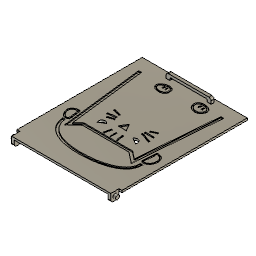
盖子 (Autodesk Fusion 360 design; units mm, degrees)
part number: 2025-10-22-10-29-16-926
Autodesk Fusion 360 part; units mm, degrees
sketch "Sketch1" plane through (0, 0, 0) normal (0, 0, 1) x (1, 0, 0)
  line L0 (50.828, 64.624) -> (-50.828, 64.624)
  line L1 (-50.828, 64.624) -> (-50.828, -64.624)
  line L2 (-50.828, -64.624) -> (50.828, -64.624)
  line L3 (50.828, -64.624) -> (50.828, 64.624)
  line L4 (50.828, 64.624) -> (-50.828, -64.624) construction
  line L5 (-50.828, 64.624) -> (50.828, -64.624) construction
  dimension "d1" = 101.656
  dimension "d2" = 129.248
  constraint horizontal L0
  constraint perpendicular L0 L1
  constraint parallel L0 L2
  constraint parallel L1 L3
  constraint coincident L4 origin
  constraint coincident L5 origin
  measures "d1" distance of L1.end L2.end
  measures "d2" distance of L0.end L1.end
extrude "Extrude1" add sketch "Sketch1" along normal blind 2
sketch "Sketch2" plane through (0, 0, 2) normal (0, 0, 1) x (-1, 0, 0)
  line L0 (-50.828, 64.624) -> (-50.828, -64.624)
  line L1 (-50.828, -64.624) -> (50.828, -64.624)
  line L2 (50.828, -64.624) -> (50.828, 64.624)
  line L3 (50.828, 64.624) -> (-50.828, 64.624)
  line L4 (0, 64.624) -> (0, -64.624) construction
  line L5 (-50.828, 64.624) -> (-48, 64.624) construction
  line L6 (-48, 64.624) -> (-48, 56.624)
  line L7 (-48, 56.624) -> (-50.828, 56.624)
  line L8 (-50.828, 56.624) -> (-50.828, 64.624) construction
  dimension "d5" = 2.828
  dimension "d6" = 8
  constraint midpoint L3 L4.start
  constraint midpoint L1 L4.end
  constraint horizontal L5
  constraint vertical L6
  constraint horizontal L7
  constraint vertical L8
  constraint coincident L0.start L3.end
  measures "d5" distance of L0.start L5.end
  measures "d6" distance of L0.start L7.end
extrude "Extrude2" cut sketch "Sketch2" against normal blind 2 contours L0 L3 L6 L7
mirror "Mirror1" about plane through (0, 0, 0) normal (1, 0, 0) of "Extrude2"
sketch "Sketch3" plane through (0, 0, 0) normal (0, 0, -1) x (1, 0, 0)
  line L0 (-48, 64.624) -> (-48, 56.624)
  line L1 (-48, 56.624) -> (-50.828, 56.624)
  line L2 (-50.828, 56.624) -> (-50.828, -64.624)
  line L3 (-50.828, -64.624) -> (50.828, -64.624)
  line L4 (50.828, -64.624) -> (50.828, 56.624)
  line L5 (50.828, 56.624) -> (48, 56.624)
  line L6 (48, 56.624) -> (48, 64.624)
  line L7 (48, 64.624) -> (-48, 64.624)
  line L8 (48, 56.624) -> (-48, 56.624)
  line L9 (-48, 56.624) -> (-48, 64.624)
  line L10 (-48, 64.624) -> (48, 64.624)
  line L11 (48, 64.624) -> (48, 56.624)
  constraint horizontal L8
  constraint vertical L9
  constraint horizontal L10
  constraint vertical L11
  constraint coincident L0.start L7.end
  constraint coincident L5.end L6.start
extrude "Extrude3" add sketch "Sketch3" along normal blind 6 contours L0 L6 L7 L8 L9 L10 L11
fillet "Fillet1" radius 2 2 edges at (0, -64.624, -6) (0, -56.624, -6)
sketch "Sketch4" plane through (48, 0, 0) normal (1, 0, 0) x (0, 1, 0)
  line L0 (-56.624, 2) -> (-64.624, 2)
  line L1 (-64.624, 2) -> (-64.624, -4)
  line L2 (-62.624, -6) -> (-58.624, -6)
  line L3 (-56.624, -4) -> (-56.624, 0)
  line L4 (-56.624, 0) -> (-56.624, 2)
  circle A0 centre (-60.624, -2) radius 1.995
  arc A1 (-58.624, -6) -> (-56.624, -4) centre (-58.624, -4) ccw
  arc A2 (-64.624, -4) -> (-62.624, -6) centre (-62.624, -4) ccw
  dimension "d13" = 3.99
  measures "d13" diameter of A0
extrude "Extrude4" add sketch "Sketch4" along normal blind 2.5 contours A0
sketch "Sketch5" plane through (0, 0, -6) normal (0, 0, -1) x (1, 0, 0)
  line L0 (-48, 62.624) -> (-48, 58.624)
  line L1 (48, 58.624) -> (48, 62.624)
  line L2 (45.3194, 56.624) -> (-45.3194, 56.624)
  line L3 (-45.3194, 56.624) -> (-45.3194, 65.376)
  line L4 (-45.3194, 65.376) -> (45.3194, 65.376)
  line L5 (45.3194, 65.376) -> (45.3194, 56.624)
  line L6 (45.3194, 56.624) -> (-45.3194, 65.376) construction
  line L7 (-45.3194, 56.624) -> (45.3194, 65.376) construction
  line L8 (-48, 58.624) -> (48, 58.624)
  line L9 (48, 62.624) -> (-48, 62.624)
  point P0 (0, 61)
  constraint horizontal L2
  constraint perpendicular L2 L3
  constraint parallel L2 L4
  constraint parallel L3 L5
  constraint coincident L6 P0
  constraint coincident L7 P0
extrude "Extrude5" cut sketch "Sketch5" against normal blind 6 contours L2 L3 L5 L8
mirror "Mirror2" about plane through (0, 0, 0) normal (1, 0, 0) of "Extrude4"
sketch "Sketch6" plane through (0, 0, -6) normal (0, 0, -1) x (1, 0, 0)
  line L0 (45.3194, 58.624) -> (48, 58.624)
  line L1 (48, 58.624) -> (48, 62.624)
  line L2 (48, 62.624) -> (-48, 62.624)
  line L3 (-48, 62.624) -> (-48, 58.624)
  line L4 (-48, 58.624) -> (-45.3194, 58.624)
  line L5 (-45.3194, 58.624) -> (45.3194, 58.624)
  line L6 (45.3194, 58.624) -> (-45.3194, 58.624)
  line L7 (-45.3194, 58.624) -> (-45.3194, 66.624)
  line L8 (-45.3194, 66.624) -> (45.3194, 66.624)
  line L9 (45.3194, 66.624) -> (45.3194, 58.624)
  line L10 (45.3194, 58.624) -> (-45.3194, 66.624) construction
  line L11 (-45.3194, 58.624) -> (45.3194, 66.624) construction
  point P0 (0, 62.624)
  constraint horizontal L6
  constraint perpendicular L6 L7
  constraint parallel L6 L8
  constraint parallel L7 L9
  constraint coincident L10 P0
  constraint coincident L11 P0
  constraint coincident L0.start L5.end
  constraint midpoint L2 P0
extrude "Extrude6" cut sketch "Sketch6" against normal blind 6 contours L2 L5 L6 L7 L9 | L2 L7 L8 L9
sketch "Sketch7" plane through (0, 0, 2) normal (0, 0, 1) x (-1, 0, 0)
  line L0 (48, 56.624) -> (48, 64.624)
  line L1 (48, 64.624) -> (-48, 64.624)
  line L2 (-48, 64.624) -> (-48, 56.624)
  line L3 (-48, 56.624) -> (-50.828, 56.624)
  line L4 (-50.828, 56.624) -> (-50.828, -64.624)
  line L5 (-50.828, -64.624) -> (50.828, -64.624)
  line L6 (50.828, -64.624) -> (50.828, 56.624)
  line L7 (50.828, 56.624) -> (48, 56.624)
  line L8 (-39.5943, -52.7414) -> (-32.6577, 29.4135)
  line L9 (-32.6577, 29.4135) -> (-22.0361, 21.1764)
  line L10 (-22.0361, 21.1764) -> (23.0515, 21.1764)
  line L11 (23.0515, 21.1764) -> (31.7222, 29.4135)
  line L12 (31.7222, 29.4135) -> (41.26, -51.4408)
  line L13 (-36.9696, -52.963) -> (-30.4409, 24.361)
  line L14 (-30.4409, 24.361) -> (-22.9378, 18.5423)
  line L15 (-22.9378, 18.5423) -> (24.1033, 18.5423)
  line L16 (24.1033, 18.5423) -> (29.7226, 23.8806)
  line L17 (29.7226, 23.8806) -> (38.6441, -51.7494)
  line L18 (-39.5943, -52.7414) -> (-36.9696, -52.963)
  line L19 (38.6441, -51.7494) -> (41.26, -51.4408)
  line L20 (-2.9359, 4.5075) -> (5, 4.5075)
  line L21 (5, 4.5075) -> (1.0321, -2.1031)
  line L22 (1.0321, -2.1031) -> (-2.9359, 4.5075)
  line L23 (-18.3094, 10.9644) -> (-12.3137, 7.7359)
  line L24 (12.7451, 8.0434) -> (18.2795, 11.4256)
  arc A0 (-18.3094, 10.9644) -> (-12.3137, 7.7359) centre (-15.3116, 9.3501) ccw
  arc A1 (12.7451, 8.0434) -> (18.2795, 11.4256) centre (15.5123, 9.7345) ccw
  line L25 (-22.8155, 3.2022) -> (-12.8166, -0.1308)
  line L26 (-21.9822, -3.4637) -> (-13.3165, -3.4637)
  line L27 (-20.3157, -9.1297) -> (-14.8164, -6.4634)
  line L28 (12.5139, 0.0359) -> (18.1799, 2.0357)
  line L29 (13.1805, -2.4638) -> (21.1796, -1.2973)
  line L30 (13.6804, -4.9636) -> (20.513, -6.4634)
  spline S0 degree 5 poles (-22.9821, -52.7915) (-23.1909, -52.6842) (-23.5816, -52.4606) (-24.0826, -52.1018) (-24.576, -51.5819) (-24.9263, -50.8599) (-25.0487, -50.0603) (-24.9733, -49.1897) (-24.6992, -48.2825) (-24.2083, -47.3928) (-23.4823, -46.5871) (-22.5171, -45.9363) (-21.342, -45.5076) (-20.0225, -45.3576) (-18.6464, -45.5259) (-17.3154, -46.0283) (-16.1343, -46.85) (-15.2012, -47.9381) (-14.5975, -49.1937) (-14.3825, -50.4909) (-14.5879, -51.6973) (-15.2124, -52.6947) (-16.2155, -53.3978) (-17.5091, -53.7784) (-18.9717, -53.8557) (-20.4675, -53.6785) (-21.5848, -53.3838) (-22.3286, -53.1046) (-22.7733, -52.8988) (-22.9821, -52.7915) knots 0 0 0 0 0 0 0.04 0.08 0.12 0.16 0.2 0.24 0.28 0.32 0.36 0.4 0.44 0.48 0.52 0.56 0.6 0.64 0.68 0.72 0.76 0.8 0.84 0.88 0.92 0.96 1 1 1 1 1 1
  spline S1 degree 5 poles (11.6806, -52.1249) (11.4571, -52.0353) (11.039, -51.8245) (10.5044, -51.4186) (9.9867, -50.7275) (9.644, -49.72) (9.5593, -48.6839) (9.6796, -47.7229) (9.9662, -46.9053) (10.4094, -46.2496) (11.0126, -45.7464) (11.7825, -45.3744) (12.7162, -45.1189) (13.7913, -44.9862) (14.9678, -44.9933) (16.1882, -45.1621) (17.378, -45.5109) (18.4468, -46.0473) (19.2862, -46.7601) (19.7879, -47.62) (19.8641, -48.5812) (19.4664, -49.5837) (18.6094, -50.5536) (17.3805, -51.4067) (15.9117, -52.0598) (14.3588, -52.44) (13.1746, -52.4844) (12.38, -52.3622) (11.9041, -52.2145) (11.6806, -52.1249) knots 0 0 0 0 0 0 0.04 0.08 0.12 0.16 0.2 0.24 0.28 0.32 0.36 0.4 0.44 0.48 0.52 0.56 0.6 0.64 0.68 0.72 0.76 0.8 0.84 0.88 0.92 0.96 1 1 1 1 1 1
  spline S2 degree 3 poles (11.2154, -53.2851) (10.1891, -52.8736) (9.3812, -52.0952) (8.9287, -51.2214) (8.3511, -50.1058) (8.2693, -48.9088) (8.4279, -47.8741) (8.5923, -46.8016) (9.0621, -45.8338) (9.8205, -45.1515) (10.7113, -44.3499) (11.874, -43.9685) (13.1906, -43.8196) (14.6835, -43.6506) (16.4477, -43.8051) (18.0295, -44.4868) (19.0286, -44.9174) (19.9643, -45.5592) (20.5382, -46.5227) (20.9518, -47.2172) (21.1279, -48.1015) (20.9526, -48.9383) (20.6952, -50.1674) (19.8008, -51.2026) (18.6612, -51.993) (16.54, -53.4644) (13.4667, -54.1879) (11.2154, -53.2851) knots 0 0 0 0 0.081939 0.081939 0.081939 0.186549 0.186549 0.186549 0.294968 0.294968 0.294968 0.422324 0.422324 0.422324 0.566743 0.566743 0.566743 0.657963 0.657963 0.657963 0.723707 0.723707 0.723707 0.820264 0.820264 0.820264 1 1 1 1
  spline S3 degree 3 poles (-23.618, -54.0288) (-24.6321, -53.5076) (-25.4512, -52.8096) (-25.9214, -51.918) (-26.3785, -51.051) (-26.4708, -50.0971) (-26.3342, -49.1764) (-26.1607, -48.0066) (-25.6061, -46.7825) (-24.5794, -45.7973) (-23.479, -44.7413) (-21.8273, -44.0438) (-20.0498, -44.0457) (-18.4067, -44.0474) (-16.6687, -44.6567) (-15.3552, -45.8026) (-14.1282, -46.873) (-13.2824, -48.3807) (-13.1232, -49.9494) (-13.0056, -51.1089) (-13.2923, -52.3202) (-14.0125, -53.2483) (-14.7306, -54.1736) (-15.8211, -54.7492) (-16.9546, -55.0029) (-18.6257, -55.377) (-20.4277, -55.1525) (-21.9392, -54.6967) (-22.5477, -54.5132) (-23.1108, -54.2894) (-23.618, -54.0288) knots 0 0 0 0 0.0968 0.0968 0.0968 0.190927 0.190927 0.190927 0.310527 0.310527 0.310527 0.438722 0.438722 0.438722 0.557218 0.557218 0.557218 0.667914 0.667914 0.667914 0.749733 0.749733 0.749733 0.831315 0.831315 0.831315 0.951586 0.951586 0.951586 1 1 1 1
  line L31 (-23.1494, 2.2004) -> (-13.1505, -1.1325)
  line L32 (-21.9822, -2.3506) -> (-13.3165, -2.3506)
  line L33 (-20.7229, -8.29) -> (-15.2235, -5.6236)
  line L34 (12.2056, 0.9092) -> (17.8717, 2.909)
  line L35 (13.0186, -1.3541) -> (21.0177, -0.1875)
  line L36 (13.4445, -6.0384) -> (20.277, -7.5382)
  line L37 (-12.8166, -0.1308) -> (-13.1505, -1.1325)
  line L38 (-22.8155, 3.2022) -> (-23.1494, 2.2004)
  line L39 (-13.3165, -2.3506) -> (-13.3165, -3.4637)
  line L40 (-21.9822, -2.3506) -> (-21.9822, -3.4637)
  line L41 (-15.2235, -5.6236) -> (-14.8164, -6.4634)
  line L42 (-20.7229, -8.29) -> (-20.3157, -9.1297)
  line L43 (17.8717, 2.909) -> (18.1799, 2.0357)
  line L44 (12.2056, 0.9092) -> (12.5139, 0.0359)
  line L45 (13.0186, -1.3541) -> (13.1805, -2.4638)
  line L46 (13.6804, -4.9636) -> (13.4445, -6.0384)
  line L47 (20.513, -6.4634) -> (20.277, -7.5382)
  line L48 (21.0177, -0.1875) -> (21.1796, -1.2973)
  line L49 (-7, 17) -> (-6.0248, 10.3131)
  line L50 (0.3601, 17) -> (0.3601, 11)
  line L51 (7, 17) -> (5.4476, 10.3439)
  line L52 (6.0438, 17.223) -> (4.4914, 10.5669)
  line L53 (-5.9422, 17.1543) -> (-4.9671, 10.4674)
  line L54 (-0.3601, 17) -> (-0.3601, 11)
  line L55 (-0.3601, 17) -> (0.3601, 17)
  line L56 (-0.3601, 11) -> (0.3601, 11)
  line L57 (6.0438, 17.223) -> (7, 17)
  line L58 (4.4914, 10.5669) -> (5.4476, 10.3439)
  line L59 (-7, 17) -> (-5.9422, 17.1543)
  line L60 (-6.0248, 10.3131) -> (-4.9671, 10.4674)
  spline S4 degree 5 poles (-35.6583, 21.5031) (-35.6382, 21.2747) (-35.6175, 20.79) (-35.6416, 19.9829) (-35.7623, 18.7701) (-35.9904, 17.1109) (-36.2225, 15.4073) (-36.396, 13.761) (-36.4737, 12.2657) (-36.4561, 10.9952) (-36.3983, 9.9919) (-36.4181, 9.2569) (-36.6442, 8.7697) (-37.1758, 8.5026) (-38.0253, 8.4401) (-39.1167, 8.5824) (-40.3268, 8.9348) (-41.5159, 9.5012) (-42.5593, 10.2767) (-43.3857, 11.2382) (-43.9766, 12.3468) (-44.3458, 13.5544) (-44.527, 14.8101) (-44.5568, 16.0656) (-44.4604, 17.2817) (-44.2369, 18.4338) (-43.8719, 19.507) (-43.3471, 20.4921) (-42.6515, 21.3812) (-41.7915, 22.1639) (-40.8032, 22.8222) (-39.7456, 23.3319) (-38.69, 23.664) (-37.7104, 23.7866) (-36.8738, 23.6669) (-36.2298, 23.2718) (-35.8912, 22.7156) (-35.7385, 22.1603) (-35.6785, 21.7315) (-35.6583, 21.5031) knots 0 0 0 0 0 0 0.028571 0.057143 0.085714 0.114286 0.142857 0.171429 0.2 0.228571 0.257143 0.285714 0.314286 0.342857 0.371429 0.4 0.428571 0.457143 0.485714 0.514286 0.542857 0.571429 0.6 0.628571 0.657143 0.685714 0.714286 0.742857 0.771429 0.8 0.828571 0.857143 0.885714 0.914286 0.942857 0.971429 1 1 1 1 1 1
  spline S5 degree 5 poles (34.8518, 21.945) (34.7664, 21.7612) (34.6267, 21.3657) (34.5096, 20.6933) (34.5218, 19.6611) (34.7263, 18.2148) (35.0077, 16.6911) (35.2626, 15.1718) (35.4246, 13.7375) (35.4956, 12.4614) (35.5694, 11.4052) (35.7794, 10.6158) (36.251, 10.1229) (37.0546, 9.9359) (38.1528, 10.0401) (39.431, 10.404) (40.7346, 10.9863) (41.9049, 11.7438) (42.8126, 12.6378) (43.3986, 13.643) (43.6617, 14.7424) (43.6362, 15.9211) (43.3734, 17.159) (42.9223, 18.4255) (42.3078, 19.6714) (41.5406, 20.8348) (40.6282, 21.8488) (39.5876, 22.6474) (38.455, 23.1732) (37.3009, 23.3842) (36.2321, 23.2594) (35.5341, 22.8896) (35.1387, 22.4685) (34.9371, 22.1288) (34.8518, 21.945) knots 0 0 0 0 0 0 0.033333 0.066667 0.1 0.133333 0.166667 0.2 0.233333 0.266667 0.3 0.333333 0.366667 0.4 0.433333 0.466667 0.5 0.533333 0.566667 0.6 0.633333 0.666667 0.7 0.733333 0.766667 0.8 0.833333 0.866667 0.9 0.933333 0.966667 1 1 1 1 1 1
  spline S6 degree 5 poles (-39.4847, 25.2158) (-39.5154, 26.2725) (-39.4254, 28.3267) (-38.836, 31.2302) (-37.135, 34.7436) (-33.4717, 38.5201) (-28.3084, 41.6536) (-21.7746, 44.1099) (-14.1533, 45.8544) (-5.8392, 46.8513) (2.7148, 47.0639) (11.041, 46.4564) (18.7049, 44.9989) (25.3459, 42.6719) (30.7407, 39.4783) (34.7923, 35.4391) (36.9395, 31.5511) (37.9405, 28.275) (38.3388, 25.9321) (38.4708, 24.7209) knots 0 0 0 0 0 0 0.066667 0.133333 0.2 0.266667 0.333333 0.4 0.466667 0.533333 0.6 0.666667 0.733333 0.8 0.866667 0.933333 1 1 1 1 1 1
  spline S7 degree 3 poles (35.8734, 21.4706) (35.7031, 21.1039) (35.6254, 20.438) (35.705, 19.5509) (35.822, 18.2465) (36.2066, 16.536) (36.4063, 14.9697) (36.604, 13.4192) (36.6239, 11.9788) (36.7576, 11.4443) (36.8125, 11.2247) (36.8524, 11.1997) (36.8529, 11.1993) (36.8533, 11.1989) (36.8884, 11.1596) (37.0973, 11.1395) (37.4923, 11.1015) (38.3785, 11.2459) (39.2583, 11.596) (40.1738, 11.9604) (41.0618, 12.5139) (41.6092, 13.0878) (42.3015, 13.8135) (42.5361, 14.5294) (42.4838, 15.504) (42.3927, 17.2008) (41.2717, 19.6563) (39.7975, 20.9993) (38.9924, 21.7328) (38.0595, 22.1367) (37.3072, 22.1736) (36.7832, 22.1993) (36.3986, 22.0631) (36.1625, 21.8614) (36.0464, 21.7622) (35.9536, 21.6433) (35.8734, 21.4706) knots 0 0 0 0 0.070845 0.070845 0.070845 0.175024 0.175024 0.175024 0.278146 0.278146 0.278146 0.320511 0.320511 0.320511 0.361672 0.361672 0.361672 0.439521 0.439521 0.439521 0.520538 0.520538 0.520538 0.622989 0.622989 0.622989 0.801373 0.801373 0.801373 0.898789 0.898789 0.898789 0.966648 0.966648 0.966648 1 1 1 1
  spline S8 degree 3 poles (-36.7923, 21.403) (-36.7005, 20.3624) (-36.9531, 18.5226) (-37.2049, 16.613) (-37.4241, 14.9507) (-37.5881, 13.2404) (-37.5948, 11.8984) (-37.5994, 10.9934) (-37.5466, 10.2421) (-37.5573, 9.8376) (-37.5594, 9.7619) (-37.5634, 9.6985) (-37.5684, 9.6508) knots 0 0 0 0 0.096531 0.096531 0.096531 0.180562 0.180562 0.180562 0.237224 0.237224 0.237224 0.247833 0.247833 0.247833 0.247833
  spline S9 degree 3 poles (-37.5684, 9.6508) (-37.6994, 9.627) (-37.9451, 9.6147) (-38.2489, 9.6433) (-39.0218, 9.7161) (-40.1374, 10.0478) (-40.9945, 10.5917) (-42.1352, 11.3156) (-42.8404, 12.3867) (-43.1625, 13.7071) (-43.4961, 15.0748) (-43.4532, 16.6591) (-43.1475, 17.9384) (-42.8802, 19.0573) (-42.3977, 19.9681) (-41.6198, 20.7419) (-40.886, 21.4718) (-39.8483, 22.0798) (-38.9109, 22.3784) (-38.2959, 22.5743) (-37.7446, 22.6174) (-37.4474, 22.5627) (-37.2095, 22.5189) (-37.1473, 22.4731) (-37.0554, 22.3497) (-36.9626, 22.225) (-36.839, 21.9314) (-36.7923, 21.403) knots 0.318735 0.318735 0.318735 0.318735 0.350635 0.350635 0.350635 0.431806 0.431806 0.431806 0.539847 0.539847 0.539847 0.651751 0.651751 0.651751 0.749617 0.749617 0.749617 0.841932 0.841932 0.841932 0.902503 0.902503 0.902503 0.950987 0.950987 0.950987 1 1 1 1
  spline S10 degree 3 poles (-37.2774, 25.28) (-37.3708, 28.4905) (-36.5566, 31.1514) (-34.7789, 33.5483) (-33.0754, 35.8449) (-30.401, 37.909) (-26.7469, 39.6189) (-22.4736, 41.6185) (-16.8751, 43.1075) (-10.7481, 43.9282) (-3.859, 44.851) (3.6489, 44.9326) (10.3612, 44.0838) (15.7001, 43.4086) (20.511, 42.1419) (24.3484, 40.3397) (28.3419, 38.4643) (31.2853, 36.0416) (33.2588, 33.1044) (34.9078, 30.65) (35.9129, 27.8109) (36.2756, 24.4818) knots 0 0 0 0 0.137831 0.137831 0.137831 0.269899 0.269899 0.269899 0.42435 0.42435 0.42435 0.598011 0.598011 0.598011 0.73614 0.73614 0.73614 0.879885 0.879885 0.879885 1 1 1 1
  line L61 (36.2756, 24.4818) -> (38.4708, 24.7209)
  line L62 (-39.4847, 25.2158) -> (-37.2774, 25.28)
  line L63 (-21.1705, -49.6333) -> (-21.1705, -52.1249)
  line L64 (-17.5048, -50.1332) -> (-18.4212, -52.7159)
  line L65 (13, -49) -> (13, -51.2996)
  line L66 (16, -49) -> (15.4038, -51.1329)
  line L67 (-18.3918, -49.8184) -> (-19.3082, -52.4011)
  line L68 (-22.1292, -49.6333) -> (-22.1292, -52.1249)
  line L69 (12.3797, -49) -> (12.3797, -51.2996)
  line L70 (15.0962, -48.7474) -> (14.5, -50.8803)
  line L71 (-18.3918, -49.8184) -> (-17.5048, -50.1332)
  line L72 (-18.4212, -52.7159) -> (-19.3082, -52.4011)
  line L73 (-21.1705, -49.6333) -> (-22.1292, -49.6333)
  line L74 (-22.1292, -52.1249) -> (-21.1705, -52.1249)
  line L75 (12.3797, -49) -> (13, -49)
  line L76 (13, -51.2996) -> (12.3797, -51.2996)
  line L77 (15.0962, -48.7474) -> (16, -49)
  line L78 (15.4038, -51.1329) -> (14.5, -50.8803)
  point P0 (-25, -50)
  point P1 (-22.9821, -46.2922)
  point P2 (-16.1496, -46.9588)
  point P3 (-15.483, -52.7915)
  point P4 (9.6809, -47.9587)
  point P5 (11.6806, -45.459)
  point P6 (17.5133, -45.6256)
  point P7 (19.5131, -49.2919)
  point P8 (-36.4502, 11.2089)
  point P9 (-36.9253, 8.675)
  point P10 (-41.8348, 9.7836)
  point P11 (-44.5272, 15.9601)
  point P12 (-42.4683, 21.5031)
  point P13 (-37.5588, 23.7203)
  point P14 (35.3902, 13.9129)
  point P15 (36.3902, 10.1706)
  point P16 (42.0173, 11.925)
  point P17 (43.2842, 17.3096)
  point P18 (38.7538, 22.9855)
  point P19 (-27.1742, 41.8521)
  point P20 (21.1719, 43.9707)
  dimension "d24" = 2.6341
  dimension "d25" = -1.25
  dimension "d26" = -1.3911
  dimension "d27" = 1.056
  dimension "d28" = -1.1131
  dimension "d29" = -0.9333
  dimension "d30" = -0.9261
  dimension "d31" = -1.1215
  dimension "d32" = 1.1005
  dimension "d33" = 0.9819
  dimension "d34" = -1.0689
  dimension "d35" = 0.7202
  dimension "d36" = -1.1264
  dimension "d37" = 1.1384
  dimension "d38" = 2.2082
  dimension "d40" = 0.9412
  dimension "d41" = 0.9587
  dimension "d42" = 0.6203
  dimension "d43" = 0.9385
  constraint parallel L5 L10
  constraint perpendicular L13 L18
  constraint perpendicular L12 L19
  constraint perpendicular L6 L20
  constraint horizontal L26
  constraint perpendicular L31 L37
  constraint perpendicular L31 L38
  constraint perpendicular L26 L39
  constraint perpendicular L26 L40
  constraint perpendicular L27 L41
  constraint perpendicular L27 L42
  constraint perpendicular L28 L43
  constraint perpendicular L28 L44
  constraint perpendicular L29 L45
  constraint perpendicular L36 L46
  constraint perpendicular L36 L47
  constraint perpendicular L29 L48
  constraint perpendicular L35 L49
  constraint vertical L50
  constraint perpendicular L50 L55
  constraint perpendicular L50 L56
  constraint perpendicular L51 L57
  constraint perpendicular L51 L58
  constraint perpendicular L53 L59
  constraint perpendicular L53 L60
  constraint vertical L63
  constraint vertical L65
  constraint perpendicular L64 L71
  constraint perpendicular L67 L72
  constraint perpendicular L68 L73
  constraint perpendicular L63 L74
  constraint perpendicular L65 L75
  constraint perpendicular L69 L76
  constraint perpendicular L66 L77
  constraint perpendicular L70 L78
extrude "Extrude7" cut sketch "Sketch7" against normal blind 1 contours L8 L9 L10 L11 L12 L13 L14 L15 L16 L17 L18 L19 | L20 L21 L22 | L25 L31 L37 L38 | L26 L32 L39 L40 | L27 L33 L41 L42 | L28 L34 L43 L44 | L29 L35 L45 L48 | L30 L36 L46 L47 | S2 | S3 | L49 L53 L59 L60 | L50 L54 L55 L56 | L51 L52 L57 L58 | S4 | S5 | S6 S10 L61 L62 | L63 L68 L73 L74 | L64 L67 L71 L72 | L65 L69 L75 L76 | L66 L70 L77 L78
sketch "Sketch8" plane through (0, 0, 2) normal (0, 0, 1) x (-1, 0, 0)
  spline S0 degree 5 poles (-35.6583, 21.5031) (-35.6382, 21.2747) (-35.6175, 20.79) (-35.6416, 19.9829) (-35.7623, 18.7701) (-35.9904, 17.1109) (-36.2225, 15.4073) (-36.396, 13.761) (-36.4737, 12.2657) (-36.4561, 10.9952) (-36.3983, 9.9919) (-36.4181, 9.2569) (-36.6442, 8.7697) (-37.1758, 8.5026) (-38.0253, 8.4401) (-39.1167, 8.5824) (-40.3268, 8.9348) (-41.5159, 9.5012) (-42.5593, 10.2767) (-43.3857, 11.2382) (-43.9766, 12.3468) (-44.3458, 13.5544) (-44.527, 14.8101) (-44.5568, 16.0656) (-44.4604, 17.2817) (-44.2369, 18.4338) (-43.8719, 19.507) (-43.3471, 20.4921) (-42.6515, 21.3812) (-41.7915, 22.1639) (-40.8032, 22.8222) (-39.7456, 23.3319) (-38.69, 23.664) (-37.7104, 23.7866) (-36.8738, 23.6669) (-36.2298, 23.2718) (-35.8912, 22.7156) (-35.7385, 22.1603) (-35.6785, 21.7315) (-35.6583, 21.5031) knots 0 0 0 0 0 0 0.028571 0.057143 0.085714 0.114286 0.142857 0.171429 0.2 0.228571 0.257143 0.285714 0.314286 0.342857 0.371429 0.4 0.428571 0.457143 0.485714 0.514286 0.542857 0.571429 0.6 0.628571 0.657143 0.685714 0.714286 0.742857 0.771429 0.8 0.828571 0.857143 0.885714 0.914286 0.942857 0.971429 1 1 1 1 1 1
  line L0 (-21.9822, -3.4637) -> (-21.9822, -2.3506)
  line L1 (-21.9822, -2.3506) -> (-13.3165, -2.3506)
  line L2 (-13.3165, -2.3506) -> (-13.3165, -3.4637)
  line L3 (-13.3165, -3.4637) -> (-21.9822, -3.4637)
  line L4 (5.4476, 10.3439) -> (4.4914, 10.5669)
  line L5 (4.4914, 10.5669) -> (6.0438, 17.223)
  line L6 (6.0438, 17.223) -> (7, 17)
  line L7 (7, 17) -> (5.4476, 10.3439)
  line L8 (12.5139, 0.0359) -> (12.2056, 0.9092)
  line L9 (12.2056, 0.9092) -> (17.8717, 2.909)
  line L10 (17.8717, 2.909) -> (18.1799, 2.0357)
  line L11 (18.1799, 2.0357) -> (12.5139, 0.0359)
  line L12 (21.1796, -1.2973) -> (13.1805, -2.4638)
  line L13 (13.1805, -2.4638) -> (13.0186, -1.3541)
  line L14 (13.0186, -1.3541) -> (21.0177, -0.1875)
  line L15 (21.0177, -0.1875) -> (21.1796, -1.2973)
  line L16 (0.3601, 11) -> (-0.3601, 11)
  line L17 (-0.3601, 11) -> (-0.3601, 17)
  line L18 (-0.3601, 17) -> (0.3601, 17)
  line L19 (0.3601, 17) -> (0.3601, 11)
  line L20 (-20.3157, -9.1297) -> (-20.7229, -8.29)
  line L21 (-20.7229, -8.29) -> (-15.2235, -5.6236)
  line L22 (-15.2235, -5.6236) -> (-14.8164, -6.4634)
  line L23 (-14.8164, -6.4634) -> (-20.3157, -9.1297)
  spline S1 degree 5 poles (34.8518, 21.945) (34.9371, 22.1288) (35.1387, 22.4685) (35.5341, 22.8896) (36.2321, 23.2594) (37.3009, 23.3842) (38.455, 23.1732) (39.5876, 22.6474) (40.6282, 21.8488) (41.5406, 20.8348) (42.3078, 19.6714) (42.9223, 18.4255) (43.3734, 17.159) (43.6362, 15.9211) (43.6617, 14.7424) (43.3986, 13.643) (42.8126, 12.6378) (41.9049, 11.7438) (40.7346, 10.9863) (39.431, 10.404) (38.1528, 10.0401) (37.0546, 9.9359) (36.251, 10.1229) (35.7794, 10.6158) (35.5694, 11.4052) (35.4956, 12.4614) (35.4246, 13.7375) (35.2626, 15.1718) (35.0077, 16.6911) (34.7263, 18.2148) (34.5218, 19.6611) (34.5096, 20.6933) (34.6267, 21.3657) (34.7664, 21.7612) (34.8518, 21.945) knots -1 -1 -1 -1 -1 -1 -0.966667 -0.933333 -0.9 -0.866667 -0.833333 -0.8 -0.766667 -0.733333 -0.7 -0.666667 -0.633333 -0.6 -0.566667 -0.533333 -0.5 -0.466667 -0.433333 -0.4 -0.366667 -0.333333 -0.3 -0.266667 -0.233333 -0.2 -0.166667 -0.133333 -0.1 -0.066667 -0.033333 0 0 0 0 0 0
  spline S2 degree 3 poles (11.2154, -53.2851) (10.1891, -52.8736) (9.3812, -52.0952) (8.9287, -51.2214) (8.3511, -50.1058) (8.2693, -48.9088) (8.4279, -47.8741) (8.5923, -46.8016) (9.0621, -45.8338) (9.8205, -45.1515) (10.7113, -44.3499) (11.874, -43.9685) (13.1906, -43.8196) (14.6835, -43.6506) (16.4477, -43.8051) (18.0295, -44.4868) (19.0286, -44.9174) (19.9643, -45.5592) (20.5382, -46.5227) (20.9518, -47.2172) (21.1279, -48.1015) (20.9526, -48.9383) (20.6952, -50.1674) (19.8008, -51.2026) (18.6612, -51.993) (16.54, -53.4644) (13.4667, -54.1879) (11.2154, -53.2851) knots 0 0 0 0 0.081939 0.081939 0.081939 0.186549 0.186549 0.186549 0.294968 0.294968 0.294968 0.422324 0.422324 0.422324 0.566743 0.566743 0.566743 0.657963 0.657963 0.657963 0.723707 0.723707 0.723707 0.820264 0.820264 0.820264 1 1 1 1
  line L24 (-23.1494, 2.2004) -> (-22.8155, 3.2022)
  line L25 (-22.8155, 3.2022) -> (-12.8166, -0.1308)
  line L26 (-12.8166, -0.1308) -> (-13.1505, -1.1325)
  line L27 (-13.1505, -1.1325) -> (-23.1494, 2.2004)
  line L28 (-2.9359, 4.5075) -> (5, 4.5075)
  line L29 (5, 4.5075) -> (1.0321, -2.1031)
  line L30 (1.0321, -2.1031) -> (-2.9359, 4.5075)
  line L31 (-30.4409, 24.361) -> (-36.9696, -52.963)
  line L32 (-36.9696, -52.963) -> (-39.5943, -52.7414)
  line L33 (-39.5943, -52.7414) -> (-32.6577, 29.4135)
  line L34 (-32.6577, 29.4135) -> (-22.0361, 21.1764)
  line L35 (-22.0361, 21.1764) -> (23.0515, 21.1764)
  line L36 (23.0515, 21.1764) -> (31.7222, 29.4135)
  line L37 (31.7222, 29.4135) -> (41.26, -51.4408)
  line L38 (41.26, -51.4408) -> (38.6441, -51.7494)
  line L39 (38.6441, -51.7494) -> (29.7226, 23.8806)
  line L40 (29.7226, 23.8806) -> (24.1033, 18.5423)
  line L41 (24.1033, 18.5423) -> (-22.9378, 18.5423)
  line L42 (-22.9378, 18.5423) -> (-30.4409, 24.361)
  line L43 (20.277, -7.5382) -> (13.4445, -6.0384)
  line L44 (13.4445, -6.0384) -> (13.6804, -4.9636)
  line L45 (13.6804, -4.9636) -> (20.513, -6.4634)
  line L46 (20.513, -6.4634) -> (20.277, -7.5382)
  line L47 (-4.9671, 10.4674) -> (-6.0248, 10.3131)
  line L48 (-6.0248, 10.3131) -> (-7, 17)
  line L49 (-7, 17) -> (-5.9422, 17.1543)
  line L50 (-5.9422, 17.1543) -> (-4.9671, 10.4674)
  spline S3 degree 3 poles (-23.618, -54.0288) (-24.6321, -53.5076) (-25.4512, -52.8096) (-25.9214, -51.918) (-26.3785, -51.051) (-26.4708, -50.0971) (-26.3342, -49.1764) (-26.1607, -48.0066) (-25.6061, -46.7825) (-24.5794, -45.7973) (-23.479, -44.7413) (-21.8273, -44.0438) (-20.0498, -44.0457) (-18.4067, -44.0474) (-16.6687, -44.6567) (-15.3552, -45.8026) (-14.1282, -46.873) (-13.2824, -48.3807) (-13.1232, -49.9494) (-13.0056, -51.1089) (-13.2923, -52.3202) (-14.0125, -53.2483) (-14.7306, -54.1736) (-15.8211, -54.7492) (-16.9546, -55.0029) (-18.6257, -55.377) (-20.4277, -55.1525) (-21.9392, -54.6967) (-22.5477, -54.5132) (-23.1108, -54.2894) (-23.618, -54.0288) knots 0 0 0 0 0.0968 0.0968 0.0968 0.190927 0.190927 0.190927 0.310527 0.310527 0.310527 0.438722 0.438722 0.438722 0.557218 0.557218 0.557218 0.667914 0.667914 0.667914 0.749733 0.749733 0.749733 0.831315 0.831315 0.831315 0.951586 0.951586 0.951586 1 1 1 1
  spline S4 degree 3 poles (36.2756, 24.4818) (35.9129, 27.8109) (34.9078, 30.65) (33.2588, 33.1044) (31.2853, 36.0416) (28.3419, 38.4643) (24.3484, 40.3397) (20.511, 42.1419) (15.7001, 43.4086) (10.3612, 44.0838) (3.6489, 44.9326) (-3.859, 44.851) (-10.7481, 43.9282) (-16.8751, 43.1075) (-22.4736, 41.6185) (-26.7469, 39.6189) (-30.401, 37.909) (-33.0754, 35.8449) (-34.7789, 33.5483) (-36.5566, 31.1514) (-37.3708, 28.4905) (-37.2774, 25.28) knots -1 -1 -1 -1 -0.879885 -0.879885 -0.879885 -0.73614 -0.73614 -0.73614 -0.598011 -0.598011 -0.598011 -0.42435 -0.42435 -0.42435 -0.269899 -0.269899 -0.269899 -0.137831 -0.137831 -0.137831 0 0 0 0
  line L51 (-37.2774, 25.28) -> (-39.4847, 25.2158)
  spline S5 degree 5 poles (-39.4847, 25.2158) (-39.5154, 26.2725) (-39.4254, 28.3267) (-38.836, 31.2302) (-37.135, 34.7436) (-33.4717, 38.5201) (-28.3084, 41.6536) (-21.7746, 44.1099) (-14.1533, 45.8544) (-5.8392, 46.8513) (2.7148, 47.0639) (11.041, 46.4564) (18.7049, 44.9989) (25.3459, 42.6719) (30.7407, 39.4783) (34.7923, 35.4391) (36.9395, 31.5511) (37.9405, 28.275) (38.3388, 25.9321) (38.4708, 24.7209) knots 0 0 0 0 0 0 0.066667 0.133333 0.2 0.266667 0.333333 0.4 0.466667 0.533333 0.6 0.666667 0.733333 0.8 0.866667 0.933333 1 1 1 1 1 1
  line L52 (38.4708, 24.7209) -> (36.2756, 24.4818)
  line L53 (48, 56.624) -> (48, 64.624)
  line L54 (48, 64.624) -> (-48, 64.624)
  line L55 (-48, 64.624) -> (-48, 56.624)
  line L56 (-48, 56.624) -> (-50.828, 56.624)
  line L57 (-50.828, 56.624) -> (-50.828, -64.624)
  line L58 (-50.828, -64.624) -> (50.828, -64.624)
  line L59 (50.828, -64.624) -> (50.828, 56.624)
  line L60 (50.828, 56.624) -> (48, 56.624)
  line L61 (-18.3094, 10.9644) -> (-12.3137, 7.7359)
  arc A0 (-18.3094, 10.9644) -> (-12.3137, 7.7359) centre (-15.3116, 9.3501) ccw
  line L62 (12.7451, 8.0434) -> (18.2795, 11.4256)
  arc A1 (12.7451, 8.0434) -> (18.2795, 11.4256) centre (15.5123, 9.7345) ccw
extrude "Extrude8" cut sketch "Sketch8" against normal blind 10 contours L61 A0 | L62 A1
sketch "Sketch9" plane through (0, 0, 2) normal (0, 0, 1) x (-1, 0, 0)
  line L0 (12.7451, 8.0434) -> (18.2795, 11.4256)
  arc A0 (12.7451, 8.0434) -> (18.2795, 11.4256) centre (15.5123, 9.7345) ccw
  line L1 (-18.3094, 10.9644) -> (-12.3137, 7.7359)
  arc A1 (-18.3094, 10.9644) -> (-12.3137, 7.7359) centre (-15.3116, 9.3501) ccw
  spline S0 degree 5 poles (-35.6583, 21.5031) (-35.6382, 21.2747) (-35.6175, 20.79) (-35.6416, 19.9829) (-35.7623, 18.7701) (-35.9904, 17.1109) (-36.2225, 15.4073) (-36.396, 13.761) (-36.4737, 12.2657) (-36.4561, 10.9952) (-36.3983, 9.9919) (-36.4181, 9.2569) (-36.6442, 8.7697) (-37.1758, 8.5026) (-38.0253, 8.4401) (-39.1167, 8.5824) (-40.3268, 8.9348) (-41.5159, 9.5012) (-42.5593, 10.2767) (-43.3857, 11.2382) (-43.9766, 12.3468) (-44.3458, 13.5544) (-44.527, 14.8101) (-44.5568, 16.0656) (-44.4604, 17.2817) (-44.2369, 18.4338) (-43.8719, 19.507) (-43.3471, 20.4921) (-42.6515, 21.3812) (-41.7915, 22.1639) (-40.8032, 22.8222) (-39.7456, 23.3319) (-38.69, 23.664) (-37.7104, 23.7866) (-36.8738, 23.6669) (-36.2298, 23.2718) (-35.8912, 22.7156) (-35.7385, 22.1603) (-35.6785, 21.7315) (-35.6583, 21.5031) knots 0 0 0 0 0 0 0.028571 0.057143 0.085714 0.114286 0.142857 0.171429 0.2 0.228571 0.257143 0.285714 0.314286 0.342857 0.371429 0.4 0.428571 0.457143 0.485714 0.514286 0.542857 0.571429 0.6 0.628571 0.657143 0.685714 0.714286 0.742857 0.771429 0.8 0.828571 0.857143 0.885714 0.914286 0.942857 0.971429 1 1 1 1 1 1
  line L2 (-21.9822, -3.4637) -> (-21.9822, -2.3506)
  line L3 (-21.9822, -2.3506) -> (-13.3165, -2.3506)
  line L4 (-13.3165, -2.3506) -> (-13.3165, -3.4637)
  line L5 (-13.3165, -3.4637) -> (-21.9822, -3.4637)
  line L6 (5.4476, 10.3439) -> (4.4914, 10.5669)
  line L7 (4.4914, 10.5669) -> (6.0438, 17.223)
  line L8 (6.0438, 17.223) -> (7, 17)
  line L9 (7, 17) -> (5.4476, 10.3439)
  line L10 (12.5139, 0.0359) -> (12.2056, 0.9092)
  line L11 (12.2056, 0.9092) -> (17.8717, 2.909)
  line L12 (17.8717, 2.909) -> (18.1799, 2.0357)
  line L13 (18.1799, 2.0357) -> (12.5139, 0.0359)
  line L14 (21.1796, -1.2973) -> (13.1805, -2.4638)
  line L15 (13.1805, -2.4638) -> (13.0186, -1.3541)
  line L16 (13.0186, -1.3541) -> (21.0177, -0.1875)
  line L17 (21.0177, -0.1875) -> (21.1796, -1.2973)
  line L18 (0.3601, 11) -> (-0.3601, 11)
  line L19 (-0.3601, 11) -> (-0.3601, 17)
  line L20 (-0.3601, 17) -> (0.3601, 17)
  line L21 (0.3601, 17) -> (0.3601, 11)
  line L22 (-20.3157, -9.1297) -> (-20.7229, -8.29)
  line L23 (-20.7229, -8.29) -> (-15.2235, -5.6236)
  line L24 (-15.2235, -5.6236) -> (-14.8164, -6.4634)
  line L25 (-14.8164, -6.4634) -> (-20.3157, -9.1297)
  spline S1 degree 5 poles (34.8518, 21.945) (34.9371, 22.1288) (35.1387, 22.4685) (35.5341, 22.8896) (36.2321, 23.2594) (37.3009, 23.3842) (38.455, 23.1732) (39.5876, 22.6474) (40.6282, 21.8488) (41.5406, 20.8348) (42.3078, 19.6714) (42.9223, 18.4255) (43.3734, 17.159) (43.6362, 15.9211) (43.6617, 14.7424) (43.3986, 13.643) (42.8126, 12.6378) (41.9049, 11.7438) (40.7346, 10.9863) (39.431, 10.404) (38.1528, 10.0401) (37.0546, 9.9359) (36.251, 10.1229) (35.7794, 10.6158) (35.5694, 11.4052) (35.4956, 12.4614) (35.4246, 13.7375) (35.2626, 15.1718) (35.0077, 16.6911) (34.7263, 18.2148) (34.5218, 19.6611) (34.5096, 20.6933) (34.6267, 21.3657) (34.7664, 21.7612) (34.8518, 21.945) knots -1 -1 -1 -1 -1 -1 -0.966667 -0.933333 -0.9 -0.866667 -0.833333 -0.8 -0.766667 -0.733333 -0.7 -0.666667 -0.633333 -0.6 -0.566667 -0.533333 -0.5 -0.466667 -0.433333 -0.4 -0.366667 -0.333333 -0.3 -0.266667 -0.233333 -0.2 -0.166667 -0.133333 -0.1 -0.066667 -0.033333 0 0 0 0 0 0
  spline S2 degree 3 poles (11.2154, -53.2851) (10.1891, -52.8736) (9.3812, -52.0952) (8.9287, -51.2214) (8.3511, -50.1058) (8.2693, -48.9088) (8.4279, -47.8741) (8.5923, -46.8016) (9.0621, -45.8338) (9.8205, -45.1515) (10.7113, -44.3499) (11.874, -43.9685) (13.1906, -43.8196) (14.6835, -43.6506) (16.4477, -43.8051) (18.0295, -44.4868) (19.0286, -44.9174) (19.9643, -45.5592) (20.5382, -46.5227) (20.9518, -47.2172) (21.1279, -48.1015) (20.9526, -48.9383) (20.6952, -50.1674) (19.8008, -51.2026) (18.6612, -51.993) (16.54, -53.4644) (13.4667, -54.1879) (11.2154, -53.2851) knots 0 0 0 0 0.081939 0.081939 0.081939 0.186549 0.186549 0.186549 0.294968 0.294968 0.294968 0.422324 0.422324 0.422324 0.566743 0.566743 0.566743 0.657963 0.657963 0.657963 0.723707 0.723707 0.723707 0.820264 0.820264 0.820264 1 1 1 1
  line L26 (-23.1494, 2.2004) -> (-22.8155, 3.2022)
  line L27 (-22.8155, 3.2022) -> (-12.8166, -0.1308)
  line L28 (-12.8166, -0.1308) -> (-13.1505, -1.1325)
  line L29 (-13.1505, -1.1325) -> (-23.1494, 2.2004)
  line L30 (-2.9359, 4.5075) -> (5, 4.5075)
  line L31 (5, 4.5075) -> (1.0321, -2.1031)
  line L32 (1.0321, -2.1031) -> (-2.9359, 4.5075)
  line L33 (-30.4409, 24.361) -> (-36.9696, -52.963)
  line L34 (-36.9696, -52.963) -> (-39.5943, -52.7414)
  line L35 (-39.5943, -52.7414) -> (-32.6577, 29.4135)
  line L36 (-32.6577, 29.4135) -> (-22.0361, 21.1764)
  line L37 (-22.0361, 21.1764) -> (23.0515, 21.1764)
  line L38 (23.0515, 21.1764) -> (31.7222, 29.4135)
  line L39 (31.7222, 29.4135) -> (41.26, -51.4408)
  line L40 (41.26, -51.4408) -> (38.6441, -51.7494)
  line L41 (38.6441, -51.7494) -> (29.7226, 23.8806)
  line L42 (29.7226, 23.8806) -> (24.1033, 18.5423)
  line L43 (24.1033, 18.5423) -> (-22.9378, 18.5423)
  line L44 (-22.9378, 18.5423) -> (-30.4409, 24.361)
  line L45 (20.277, -7.5382) -> (13.4445, -6.0384)
  line L46 (13.4445, -6.0384) -> (13.6804, -4.9636)
  line L47 (13.6804, -4.9636) -> (20.513, -6.4634)
  line L48 (20.513, -6.4634) -> (20.277, -7.5382)
  line L49 (-4.9671, 10.4674) -> (-6.0248, 10.3131)
  line L50 (-6.0248, 10.3131) -> (-7, 17)
  line L51 (-7, 17) -> (-5.9422, 17.1543)
  line L52 (-5.9422, 17.1543) -> (-4.9671, 10.4674)
  spline S3 degree 3 poles (-23.618, -54.0288) (-24.6321, -53.5076) (-25.4512, -52.8096) (-25.9214, -51.918) (-26.3785, -51.051) (-26.4708, -50.0971) (-26.3342, -49.1764) (-26.1607, -48.0066) (-25.6061, -46.7825) (-24.5794, -45.7973) (-23.479, -44.7413) (-21.8273, -44.0438) (-20.0498, -44.0457) (-18.4067, -44.0474) (-16.6687, -44.6567) (-15.3552, -45.8026) (-14.1282, -46.873) (-13.2824, -48.3807) (-13.1232, -49.9494) (-13.0056, -51.1089) (-13.2923, -52.3202) (-14.0125, -53.2483) (-14.7306, -54.1736) (-15.8211, -54.7492) (-16.9546, -55.0029) (-18.6257, -55.377) (-20.4277, -55.1525) (-21.9392, -54.6967) (-22.5477, -54.5132) (-23.1108, -54.2894) (-23.618, -54.0288) knots 0 0 0 0 0.0968 0.0968 0.0968 0.190927 0.190927 0.190927 0.310527 0.310527 0.310527 0.438722 0.438722 0.438722 0.557218 0.557218 0.557218 0.667914 0.667914 0.667914 0.749733 0.749733 0.749733 0.831315 0.831315 0.831315 0.951586 0.951586 0.951586 1 1 1 1
  spline S4 degree 3 poles (36.2756, 24.4818) (35.9129, 27.8109) (34.9078, 30.65) (33.2588, 33.1044) (31.2853, 36.0416) (28.3419, 38.4643) (24.3484, 40.3397) (20.511, 42.1419) (15.7001, 43.4086) (10.3612, 44.0838) (3.6489, 44.9326) (-3.859, 44.851) (-10.7481, 43.9282) (-16.8751, 43.1075) (-22.4736, 41.6185) (-26.7469, 39.6189) (-30.401, 37.909) (-33.0754, 35.8449) (-34.7789, 33.5483) (-36.5566, 31.1514) (-37.3708, 28.4905) (-37.2774, 25.28) knots -1 -1 -1 -1 -0.879885 -0.879885 -0.879885 -0.73614 -0.73614 -0.73614 -0.598011 -0.598011 -0.598011 -0.42435 -0.42435 -0.42435 -0.269899 -0.269899 -0.269899 -0.137831 -0.137831 -0.137831 0 0 0 0
  line L53 (-37.2774, 25.28) -> (-39.4847, 25.2158)
  spline S5 degree 5 poles (-39.4847, 25.2158) (-39.5154, 26.2725) (-39.4254, 28.3267) (-38.836, 31.2302) (-37.135, 34.7436) (-33.4717, 38.5201) (-28.3084, 41.6536) (-21.7746, 44.1099) (-14.1533, 45.8544) (-5.8392, 46.8513) (2.7148, 47.0639) (11.041, 46.4564) (18.7049, 44.9989) (25.3459, 42.6719) (30.7407, 39.4783) (34.7923, 35.4391) (36.9395, 31.5511) (37.9405, 28.275) (38.3388, 25.9321) (38.4708, 24.7209) knots 0 0 0 0 0 0 0.066667 0.133333 0.2 0.266667 0.333333 0.4 0.466667 0.533333 0.6 0.666667 0.733333 0.8 0.866667 0.933333 1 1 1 1 1 1
  line L54 (38.4708, 24.7209) -> (36.2756, 24.4818)
  line L55 (48, 56.624) -> (48, 64.624)
  line L56 (48, 64.624) -> (-48, 64.624)
  line L57 (-48, 64.624) -> (-48, 56.624)
  line L58 (-48, 56.624) -> (-50.828, 56.624)
  line L59 (-50.828, 56.624) -> (-50.828, -64.624)
  line L60 (-50.828, -64.624) -> (50.828, -64.624)
  line L61 (50.828, -64.624) -> (50.828, 56.624)
  line L62 (50.828, 56.624) -> (48, 56.624)
  line L63 (21.7186, -58.5) -> (-21.7186, -58.5)
  line L64 (-21.7186, -58.5) -> (-21.7186, -61.5)
  line L65 (-21.7186, -61.5) -> (21.7186, -61.5)
  line L66 (21.7186, -61.5) -> (21.7186, -58.5)
  line L67 (21.7186, -58.5) -> (-21.7186, -61.5) construction
  line L68 (-21.7186, -58.5) -> (21.7186, -61.5) construction
  point P0 (0, -60)
  dimension "d48" = 3
  constraint horizontal L63
  constraint perpendicular L63 L64
  constraint parallel L63 L65
  constraint parallel L64 L66
  constraint coincident L67 P0
  constraint coincident L68 P0
  measures "d48" distance of L63.end L64.end
extrude "Extrude9" add sketch "Sketch9" along normal blind 5 contours L63 L64 L65 L66
fillet "Fillet2" radius 2 2 edges at (21.7186, 60, 7) (-21.7186, 60, 7)
sketch "Sketch10" plane through (0, 61.5, 0) normal (0, 1, 0) x (-1, 0, 0)
  arc A0 (21.7186, 5) -> (19.7186, 7) centre (19.7186, 5) ccw
  line L0 (19.7186, 7) -> (-19.7186, 7)
  arc A1 (-19.7186, 7) -> (-21.7186, 5) centre (-19.7186, 5) ccw
  line L1 (-21.7186, 5) -> (-21.7186, 2)
  line L2 (-21.7186, 2) -> (21.7186, 2)
  line L3 (21.7186, 2) -> (21.7186, 5)
  line L4 (0, 2) -> (0, 4.5)
  line L5 (0, 4.5) -> (17, 4.5)
  line L6 (18, 3.5) -> (18, 2)
  line L7 (18, 2) -> (0, 2)
  line L8 (0, 2) -> (0, 4.5)
  line L9 (0, 4.5) -> (-17, 4.5)
  line L10 (-18, 3.5) -> (-18, 2)
  line L11 (-18, 2) -> (0, 2)
  line L12 (0, 2) -> (0, 4.5)
  arc A2 (-17, 4.5) -> (-18, 3.5) centre (-17, 3.5) ccw
  arc A3 (18, 3.5) -> (17, 4.5) centre (17, 3.5) ccw
  dimension "d53" = 2.5
  dimension "d54" = 1
  constraint midpoint L2 L4.start
  constraint perpendicular L0 L4
  constraint horizontal L5
  constraint vertical L6
  constraint horizontal L7
  constraint vertical L8
  constraint coincident L2 L6.end
  constraint horizontal L9
  constraint vertical L10
  constraint horizontal L11
  constraint vertical L12
  constraint coincident L2 L10.end
  constraint tangent L9 A2
  constraint tangent L10 A2
  constraint tangent L5 A3
  constraint tangent L6 A3
  constraint equal A2 A3
  measures "d53" distance of L4.start L4.end
  measures "d54" radius of A2
extrude "Extrude10" cut sketch "Sketch10" against normal blind 5 contours L2 L4 L5 L6 L7 L8 L12 A3 | L2 L4 L8 L9 L10 L11 L12 A2
